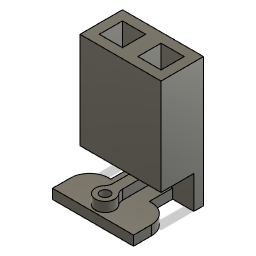
Cagacubi v1 (Autodesk Fusion 360 design; units mm, degrees)
Autodesk Fusion 360 part; units mm, degrees
sketch "Sketch1" plane through (0, 0, 0) normal (0, 1, 0) x (1, 0, 0)
  circle A0 centre (0, 0) radius 2.5
  line L0 (2.5, 6.6144) -> (2.5, 23)
  line L1 (0.5, 25) -> (-0.5, 25)
  line L2 (-2.5, 23) -> (-2.5, 6.6144)
  arc A1 (-3.75, 3.3072) -> (3.75, 3.3072) centre (0, 0) ccw
  arc A2 (-3.75, 3.3072) -> (-2.5, 6.6144) centre (-7.5, 6.6144) ccw
  arc A3 (2.5, 6.6144) -> (3.75, 3.3072) centre (7.5, 6.6144) ccw
  arc A4 (-0.5, 25) -> (-2.5, 23) centre (-0.5, 23) ccw
  arc A5 (2.5, 23) -> (0.5, 25) centre (0.5, 23) ccw
  dimension "d1" = 5
  dimension "d2" = 10
  dimension "d5" = 5
  dimension "d6" = 2
  constraint coincident A0.centre A1.centre
  constraint concentric A0 A1
  constraint vertical L0
  constraint horizontal L1
  constraint vertical L2
  constraint tangent L2 A2
  constraint tangent A1 A2
  constraint tangent A1 A3
  constraint tangent L0 A3
  constraint equal A2 A3
  constraint tangent L1 A4
  constraint tangent L2 A4
  constraint tangent L0 A5
  constraint tangent L1 A5
  constraint equal A4 A5
  measures "d1" diameter of A0
  measures "d2" diameter of A1
  measures "d5" radius of A2
  measures "d6" radius of A4
extrude "Extrude1" add sketch "Sketch1" along normal blind 5 makes body 1
sketch "Sketch5" plane through (0, 0, 0) normal (0, -1, 0) x (1, 0, 0)
  circle A0 centre (0, 0) radius 2.5
  line L0 (2.5, -23) -> (2.5, -6.6144)
  arc A1 (3.75, -3.3072) -> (2.5, -6.6144) centre (7.5, -6.6144) ccw
  arc A2 (3.75, -3.3072) -> (-3.75, -3.3072) centre (0, 0) ccw
  arc A3 (-2.5, -6.6144) -> (-3.75, -3.3072) centre (-7.5, -6.6144) ccw
  line L1 (-2.5, -6.6144) -> (-2.5, -23)
  arc A4 (-2.5, -23) -> (-0.5, -25) centre (-0.5, -23) ccw
  line L2 (-0.5, -25) -> (0.5, -25)
  arc A5 (0.5, -25) -> (2.5, -23) centre (0.5, -23) ccw
  line L3 (0, 6.25) -> (21, 6.25)
  line L4 (21, 6.25) -> (21, -30)
  line L5 (21, -30) -> (0, -30)
  line L6 (0, 6.25) -> (-21, 6.25)
  line L7 (-21, 6.25) -> (-21, -30)
  line L8 (-21, -30) -> (0, -30)
  dimension "d42" = 6.25
  dimension "d49" = 21
  dimension "d50" = 36.25
  constraint perpendicular L3 L4
  constraint perpendicular L4 L5
  measures "d42" distance of A0.centre L3.start
  measures "d49" distance of L3.start L3.end
  measures "d50" distance of L3.end L4.end
extrude "Extrude5" add sketch "Sketch5" along normal blind 5 separate body contours A0 | L0 A1 A2 A3 L1 A4 L2 A5 | L3 L4 L5 L6 L7 L8 makes body 2
sketch "Sketch6" plane through (0, 0, 0) normal (0, 1, 0) x (-1, 0, 0)
  line L0 (21, 6.25) -> (-21, 6.25)
  line L1 (-21, 6.25) -> (-21, -30)
  line L2 (-21, -30) -> (21, -30)
  line L3 (21, -30) -> (21, 6.25)
  line L4 (21, -30) -> (16, -30)
  line L5 (16, -25) -> (21, -25)
  line L6 (21, -25) -> (21, -30)
  line L7 (16, -25) -> (4, -25)
  line L8 (-4, -25) -> (-21, -25)
  arc A0 (-4, -25) -> (4, -25) centre (0, -22) ccw
  dimension "d53" = 5
  dimension "d54" = 5
  dimension "d55" = 12
  constraint horizontal L4
  constraint horizontal L5
  constraint vertical L6
  constraint coincident L2.end L3.start
  constraint horizontal L7
  constraint coincident L1 L8.end
  constraint perpendicular L1 L8
  measures "d53" distance of L2.end L4.end
  measures "d54" distance of L2.end L5.end
  measures "d55" distance of L5.start L7.end
extrude "Extrude6" add sketch "Sketch6" along normal blind 12 contours L1 L2 L3 L4 L5 L6 L7 L8 A0 bodies 2
sketch "Sketch7" plane through (0, 12, 0) normal (0, 1, 0) x (-1, 0, 0)
  line L0 (-21, -25) -> (-21, -30)
  line L1 (-21, -30) -> (21, -30)
  line L2 (21, -30) -> (21, -25)
  line L3 (21, -25) -> (4, -25)
  arc A0 (-4, -25) -> (4, -25) centre (0, -22) ccw
  line L4 (-4, -25) -> (-21, -25)
  line L5 (16, -25) -> (4, -25)
  line L6 (4, -25) -> (4, -13)
  line L7 (4, -13) -> (16, -13)
  line L8 (16, -13) -> (16, -25)
  line L9 (-16, -25) -> (-4, -25)
  line L10 (-4, -25) -> (-4, -13)
  line L11 (-4, -13) -> (-16, -13)
  line L12 (-16, -13) -> (-16, -25)
  line L13 (21, -30) -> (-21, -30)
  line L14 (-21, -30) -> (-21, -8)
  line L15 (-21, -8) -> (21, -8)
  line L16 (21, -8) -> (21, -30)
  dimension "d60" = 12
  dimension "d61" = 12
  dimension "d62" = 42
  dimension "d63" = 22
  constraint horizontal L5
  constraint vertical L6
  constraint horizontal L7
  constraint vertical L8
  constraint horizontal L13
  constraint vertical L14
  constraint horizontal L15
  constraint vertical L16
  constraint coincident L1.end L2.start
  measures "d60" distance of L5.start L3.end
  measures "d61" distance of L5.start L7.end
  measures "d62" distance of L1.end L0.end
  measures "d63" distance of L1.end L15.end
extrude "Extrude7" add sketch "Sketch7" along normal blind 50 contours L0 L1 L2 L3 A0 L4 L5 L9 L13 L14 L16 | L3 A0 L4 L6 L7 L8 L10 L11 L12 L14 L15 L16 bodies 2
sketch "Sketch8" plane through (0, 0, 0) normal (0, 1, 0) x (-1, 0, 0)
  line L0 (4, -25) -> (21, -25)
  line L1 (21, -25) -> (21, 6.25)
  line L2 (21, 6.25) -> (-21, 6.25)
  line L3 (-21, 6.25) -> (-21, -25)
  line L4 (-21, -25) -> (-4, -25)
  arc A0 (-4, -25) -> (4, -25) centre (0, -22) ccw
  line L5 (21, -25) -> (10, -25)
  line L6 (10, -25) -> (10, -13)
  line L7 (10, -13) -> (21, -13)
  line L8 (21, -13) -> (21, -25)
  line L9 (-21, -13) -> (-21, -25)
  line L10 (-21, -25) -> (-10, -25)
  line L11 (-10, -25) -> (-10, -13)
  line L12 (-10, -13) -> (-21, -13)
  constraint horizontal L5
  constraint vertical L6
  constraint horizontal L7
  constraint vertical L8
  constraint coincident L0.end L1.start
extrude "Extrude8" cut sketch "Sketch8" against normal blind 5 contours L0 L1 L5 L6 L7 L8 | L3 L4 L9 L10 L11 L12 bodies 2
fillet "Fillet1" radius 10 2 edges at (-21, -2.5, -13) (21, -2.5, -13) on bodies 2
